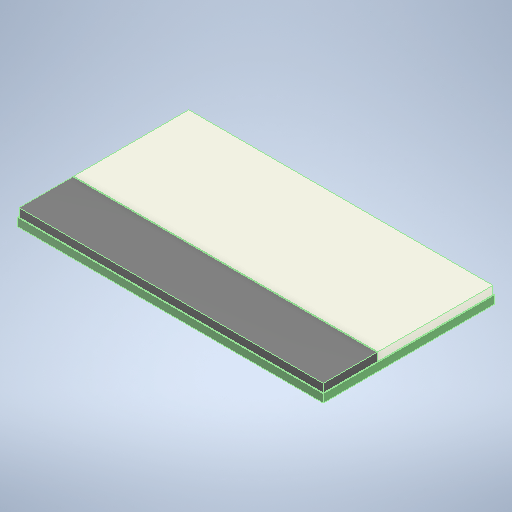
# Autodesk Inventor part: AQM1602Y
Saved by Autodesk Inventor 2025.3 (Build 293356000, 356)
## iProperties
Created: 2025-06-27
Part Number: AQM1602Y
Material: 一般
Document SubType Name: Modeling
Designer: yamashita1
Density: 1 g/cm^3
Appearance: 滑らか - 濃い深緑
Author: yamashita1
Autodesk Inventor part; units mm, degrees
ref_plane "YZ Plane" through (0, 0, 0) normal (1, 0, 0) x (0, 1, 0)
ref_plane "XZ Plane" through (0, 0, 0) normal (0, 1, 0) x (-1, 0, 0)
ref_plane "XY Plane" through (0, 0, 0) normal (0, 0, 1) x (1, 0, 0)
sketch "スケッチ1" plane through (0, 0, 0) normal (0, 0, 1) x (1, 0, 0)
  line L0 (-20.6, 23.07) -> (20.6, 23.07)
  line L1 (20.6, 23.07) -> (20.6, 0)
  line L2 (20.6, 0) -> (-20.6, 0)
  line L3 (-20.6, 0) -> (-20.6, 23.07)
  point P0 (0, 0)
  point P1 (0, 0)
  dimension "d0" = 41.2
  dimension "d1" = 23.07
  constraints: 8 end point, 2 parallel, 1 coincident, 1 horizontal, 1 midpoint, 1 perpendicular
  measures "d0" distance of L1.end L2.end
  measures "d1" distance of L0.end L1.end
extrude "押し出し1" add sketch "スケッチ1" along normal blind 1.1
sketch "スケッチ3" plane through (0, 0, 1.1) normal (0, 0, 1) x (1, 0, 0)
  line L0 (-20.5, 0.1) -> (20.5, 0.1)
  line L1 (20.5, 0.1) -> (20.5, 7.35)
  line L2 (20.5, 7.35) -> (-20.5, 7.35)
  line L3 (-20.5, 7.35) -> (-20.5, 0.1)
  line L4 (-20.6, 23.07) -> (-20.6, 0) projected
  line L5 (-20.6, 0) -> (20.6, 0) projected
  line L6 (20.6, 0) -> (20.6, 23.07) projected
  point P0 (0, 0)
  dimension "d6" = 7.25
  dimension "d7" = 0.1
  dimension "d8" = 0.1
  dimension "d9" = 0.1
  constraints: 8 end point, 2 parallel, 1 horizontal, 1 perpendicular
  measures "d6" distance of L0.end L1.end
  measures "d7" distance between parallel lines of L4 L3
  measures "d8" distance between parallel lines of L5 L0
  measures "d9" distance between parallel lines of L6 L1
extrude "押し出し2" add sketch "スケッチ3" along normal blind 1.1
sketch "スケッチ4" plane through (0, 0, 1.1) normal (0, 0, 1) x (1, 0, 0)
  line L0 (-20.5, 22.97) -> (20.5, 22.97)
  line L1 (20.5, 22.97) -> (20.5, 7.45)
  line L2 (20.5, 7.45) -> (-20.5, 7.45)
  line L3 (-20.5, 7.45) -> (-20.5, 22.97)
  line L4 (20.6, 23.07) -> (-20.6, 23.07) projected
  line L5 (20.5, 7.35) -> (-20.5, 7.35) projected
  line L6 (-20.5, 7.35) -> (-20.5, 0.1) projected
  line L7 (20.5, 0.1) -> (20.5, 7.35) projected
  point P0 (0, 0)
  dimension "d12" = 0.1
  dimension "d13" = 0.1
  constraints: 8 end point, 2 collinear, 2 parallel, 1 horizontal, 1 perpendicular
  measures "d12" distance between parallel lines of L4 L0
  measures "d13" distance between parallel lines of L5 L2
extrude "押し出し3" add sketch "スケッチ4" along normal blind 1.1
equation "\"d8\" = d7"
equation "\"d9\" = d7"
equation "\"d13\" = d12"
